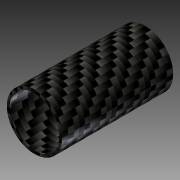
# Autodesk Inventor part: carbon-fiber-forearm
Saved by Autodesk Inventor 2016 (Build 200138000, 138)
## iProperties
Created: 2015-10-08
Part Number: carbon-fiber-forearm
Material: Generic
Document SubType Name: Modeling
Designer: eedoga
Density: 1 g/cm^3
Appearance: Carbon Fiber 1
Author: eedoga
Autodesk Inventor part; units mm, degrees
ref_plane "YZ Plane" through (0, 0, 0) normal (1, 0, 0) x (0, 1, 0)
ref_plane "XZ Plane" through (0, 0, 0) normal (0, 1, 0) x (-1, 0, 0)
ref_plane "XY Plane" through (0, 0, 0) normal (0, 0, 1) x (1, 0, 0)
sketch "Sketch1" plane through (0, 0, 0) normal (0, 0, 1) x (1, 0, 0)
  circle A0 centre (0, 0) radius 13.97 projected
  circle A1 centre (0, 0) radius 12.7
  circle A2 centre (0, 0) radius 11.43
  point P0 (0, 0)
  dimension "d0" = 25.4
  dimension "d1" = 22.86
  constraints: 2 centre point, 2 coincident
  measures "d0" diameter of A1
  measures "d1" diameter of A2
extrude "Extrusion1" add sketch "Sketch1" along normal blind 50.8 contours A1
body "Solid1"
